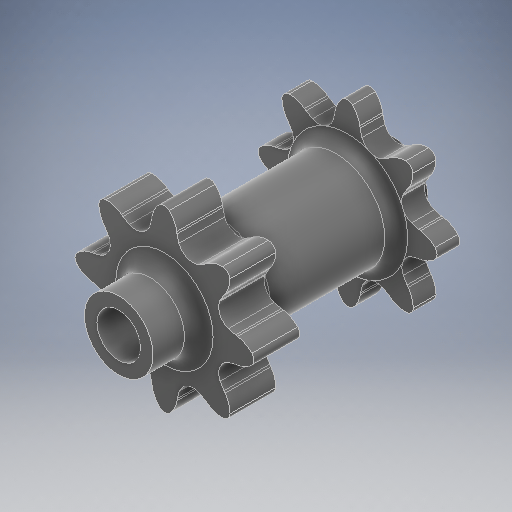
# Autodesk Inventor part: 6PSprocketElongated
Saved by Autodesk Inventor 2026.1 (Build 301233000, 233)
## iProperties
Created: 2025-10-13
Part Number: 6PSprocketElongated
Material: Plastic, Opaque Black
Document SubType Name: Modeling
Designer: Teddy
Density: 0.952 g/cm^3
Appearance: Smooth - Black
Author: Teddy
Autodesk Inventor part; units mm, degrees
ref_plane "YZ Plane" through (0, 0, 0) normal (1, 0, 0) x (0, 1, 0)
ref_plane "XZ Plane" through (0, 0, 0) normal (0, 1, 0) x (-1, 0, 0)
ref_plane "XY Plane" through (0, 0, 0) normal (0, 0, 1) x (1, 0, 0)
sketch "Sketch1" plane through (0, 0, 0) normal (0, 0, 1) x (1, 0, 0)
  spline S0 degree 3 poles (4.5605, -0.4358) (4.5398, -0.5666) (4.5107, -0.6964) (4.3363, -1.2739) (4.0837, -1.6899) (3.7565, -2.02) (3.7485, -2.028) (3.7404, -2.036) knots 0 0 0 0 0.215998 0.215998 0.980932 0.980932 1 1 1 1
  spline S1 degree 3 poles (3.7404, -2.036) (3.6739, -2.1011) (3.5927, -2.1577) (3.4009, -2.2429) (3.2878, -2.2658) (3.0745, -2.2664) (2.9612, -2.2441) (2.769, -2.1599) (2.6875, -2.1038) (2.6206, -2.039) knots 0 0 0 0 0.231931 0.231931 0.5 0.5 0.768069 0.768069 1 1 1 1
  spline S2 degree 3 poles (2.6206, -2.039) (2.6125, -2.0311) (2.6044, -2.0231) (2.2754, -1.6948) (2.0207, -1.2801) (1.8431, -0.7036) (1.8133, -0.5739) (1.7919, -0.4433) knots 0 0 0 0 0.019068 0.019068 0.784002 0.784002 1 1 1 1
  line L0 (1.7919, -0.4433) -> (1.757, -0.2271)
  spline S3 degree 3 poles (1.757, -0.2271) (1.7125, 0.0474) (1.6406, 0.3168) (1.549, 0.5685) knots 0 0 0 0 1 1 1 1
  ellipse E0 centre (-0.0213, 0.0205) end of major axis (-1.6252, 0.4958) minor radius 1.645 (1.549, 0.5685) -> (1.4956, 0.6969) ccw
  spline S4 degree 3 poles (1.4956, 0.6969) (1.4886, 0.712) (1.4813, 0.727) (1.4457, 0.7976) (1.4144, 0.852) (1.3798, 0.9048) knots 0 0 0 0 0.212597 0.212597 1 1 1 1
  arc A0 (1.3798, 0.9048) -> (-0.3446, 1.6136) centre (0, 0) ccw
  spline S5 degree 3 poles (-0.3446, 1.6136) (-0.4235, 1.5968) (-0.4998, 1.5744) (-0.5732, 1.5473) knots 0 0 0 0 1 1 1 1
  spline S6 degree 3 poles (-0.7014, 1.4935) (-0.9435, 1.3789) (-1.1841, 1.238) (-1.4088, 1.0742) knots 0 0 0 0 1 1 1 1
  ellipse E1 centre (0.0296, -0.0004) end of major axis (-1.4449, 0.7896) minor radius 1.645 (-0.5732, 1.5473) -> (-0.7014, 1.4935) ccw
  line L1 (-1.4088, 1.0742) -> (-1.5856, 0.945)
  spline S7 degree 3 poles (-1.5856, 0.945) (-1.6928, 0.8673) (-1.8052, 0.796) (-2.3368, 0.511) (-2.8095, 0.3954) (-3.2744, 0.3934) (-3.2857, 0.3934) (-3.297, 0.3935) knots 0 0 0 0 0.215998 0.215998 0.980932 0.980932 1 1 1 1
  spline S8 degree 3 poles (-3.297, 0.3935) (-3.3901, 0.3944) (-3.4875, 0.4119) (-3.6834, 0.4872) (-3.7796, 0.551) (-3.9308, 0.7015) (-3.9951, 0.7973) (-4.0715, 0.9927) (-4.0895, 1.0901) (-4.091, 1.1832) knots 0 0 0 0 0.231931 0.231931 0.5 0.5 0.768069 0.768069 1 1 1 1
  spline S9 degree 3 poles (-4.091, 1.1832) (-4.0911, 1.1945) (-4.0912, 1.2058) (-4.0917, 1.6706) (-3.9786, 2.144) (-3.6965, 2.6771) (-3.6258, 2.7899) (-3.5487, 2.8975) knots 0 0 0 0 0.019068 0.019068 0.784002 0.784002 1 1 1 1
  line L2 (-3.5487, 2.8975) -> (-3.4204, 3.075)
  spline S10 degree 3 poles (-3.4204, 3.075) (-3.2578, 3.3006) (-3.1182, 3.5419) (-3.0049, 3.7847) knots 0 0 0 0 1 1 1 1
  ellipse E2 centre (-4.5028, 4.5076) end of major axis (-5.3008, 5.9778) minor radius 1.645 (-3.0049, 3.7847) -> (-2.9519, 3.9132) ccw
  spline S11 degree 3 poles (-2.9519, 3.9132) (-2.9462, 3.9288) (-2.9407, 3.9446) (-2.9159, 4.0197) (-2.8996, 4.0803) (-2.8868, 4.1421) knots 0 0 0 0 0.212597 0.212597 1 1 1 1
  arc A1 (-2.8868, 4.1421) -> (-3.6049, 5.8627) centre (-4.5022, 4.478) ccw
  spline S12 degree 3 poles (-3.6049, 5.8627) (-3.6726, 5.9066) (-3.7424, 5.9447) (-3.8134, 5.9774) knots 0 0 0 0 1 1 1 1
  ellipse E3 centre (-4.4816, 4.4568) end of major axis (-4.9656, 6.058) minor radius 1.645 (-3.8134, 5.9774) -> (-3.9421, 6.03) ccw
  spline S13 degree 3 poles (-3.9421, 6.03) (-4.1943, 6.1202) (-4.4641, 6.1907) (-4.7388, 6.2338) knots 0 0 0 0 1 1 1 1
  line L3 (-4.7388, 6.2338) -> (-4.9552, 6.2674)
  spline S14 degree 3 poles (-4.9552, 6.2674) (-5.0859, 6.2882) (-5.2158, 6.3173) (-5.7932, 6.4917) (-6.2093, 6.7442) (-6.5394, 7.0715) (-6.5474, 7.0795) (-6.5553, 7.0876) knots 0 0 0 0 0.215998 0.215998 0.980932 0.980932 1 1 1 1
  spline S15 degree 3 poles (-6.5553, 7.0876) (-6.6205, 7.1541) (-6.677, 7.2353) (-6.7622, 7.427) (-6.7852, 7.5402) (-6.7857, 7.7535) (-6.7634, 7.8668) (-6.6793, 8.059) (-6.6232, 8.1405) (-6.5584, 8.2074) knots 0 0 0 0 0.231931 0.231931 0.5 0.5 0.768069 0.768069 1 1 1 1
  spline S16 degree 3 poles (-6.5584, 8.2074) (-6.5505, 8.2155) (-6.5425, 8.2235) (-6.2142, 8.5525) (-5.7995, 8.8073) (-5.223, 8.9848) (-5.0933, 9.0146) (-4.9627, 9.0361) knots 0 0 0 0 0.019068 0.019068 0.784002 0.784002 1 1 1 1
  line L4 (-4.9627, 9.0361) -> (-4.7465, 9.071)
  spline S17 degree 3 poles (-4.7465, 9.071) (-4.472, 9.1155) (-4.2026, 9.1874) (-3.9509, 9.279) knots 0 0 0 0 1 1 1 1
  ellipse E4 centre (-4.4988, 10.8493) end of major axis (-4.0235, 12.4532) minor radius 1.645 (-3.9509, 9.279) -> (-3.8225, 9.3324) ccw
  spline S18 degree 3 poles (-3.8225, 9.3324) (-3.7961, 9.3446) (-3.7696, 9.3578) (-3.6993, 9.3954) (-3.6564, 9.4208) (-3.6146, 9.4482) knots 0 0 0 0 0.378322 0.378322 1 1 1 1
  arc A2 (-3.6146, 9.4482) -> (-2.9058, 11.1726) centre (-4.5194, 10.828) ccw
  spline S19 degree 3 poles (-2.9058, 11.1726) (-2.9227, 11.2521) (-2.9451, 11.3283) (-2.9721, 11.4011) knots 0 0 0 0 1 1 1 1
  ellipse E5 centre (-4.5198, 10.7984) end of major axis (-3.7297, 12.2729) minor radius 1.645 (-2.9721, 11.4011) -> (-3.0258, 11.5293) ccw
  spline S20 degree 3 poles (-3.0258, 11.5293) (-3.1404, 11.7715) (-3.2813, 12.012) (-3.4451, 12.2368) knots 0 0 0 0 1 1 1 1
  line L5 (-3.4451, 12.2368) -> (-3.5743, 12.4136)
  spline S21 degree 3 poles (-3.5743, 12.4136) (-3.6521, 12.5207) (-3.7234, 12.6331) (-4.0083, 13.1648) (-4.124, 13.6375) (-4.126, 14.1023) (-4.126, 14.1136) (-4.1259, 14.125) knots 0 0 0 0 0.215998 0.215998 0.980932 0.980932 1 1 1 1
  spline S22 degree 3 poles (-4.1259, 14.125) (-4.125, 14.2181) (-4.1075, 14.3155) (-4.0321, 14.5113) (-3.9684, 14.6075) (-3.8179, 14.7588) (-3.722, 14.8231) (-3.5266, 14.8995) (-3.4293, 14.9175) (-3.3362, 14.9189) knots 0 0 0 0 0.231931 0.231931 0.5 0.5 0.768069 0.768069 1 1 1 1
  spline S23 degree 3 poles (-3.3362, 14.9189) (-3.3249, 14.9191) (-3.3136, 14.9192) (-2.8487, 14.9196) (-2.3754, 14.8066) (-1.8422, 14.5245) (-1.7294, 14.4538) (-1.6219, 14.3766) knots 0 0 0 0 0.019068 0.019068 0.784002 0.784002 1 1 1 1
  line L6 (-1.6219, 14.3766) -> (-1.4443, 14.2484)
  spline S24 degree 3 poles (-1.4443, 14.2484) (-1.2187, 14.0858) (-0.9774, 13.9462) (-0.7347, 13.8329) knots 0 0 0 0 1 1 1 1
  ellipse E6 centre (-0.0118, 15.3308) end of major axis (1.4584, 16.1288) minor radius 1.645 (-0.7347, 13.8329) -> (-0.6062, 13.7799) ccw
  spline S25 degree 3 poles (-0.6062, 13.7799) (-0.5905, 13.7742) (-0.5747, 13.7687) (-0.4996, 13.7439) (-0.439, 13.7276) (-0.3773, 13.7147) knots 0 0 0 0 0.212597 0.212597 1 1 1 1
  arc A3 (-0.3773, 13.7147) -> (1.3433, 14.4329) centre (-0.0414, 15.3302) ccw
  spline S26 degree 3 poles (1.3433, 14.4329) (1.3872, 14.5006) (1.4253, 14.5704) (1.458, 14.6414) knots 0 0 0 0 1 1 1 1
  ellipse E7 centre (-0.0626, 15.3096) end of major axis (1.5387, 15.7935) minor radius 1.645 (1.458, 14.6414) -> (1.5106, 14.7701) ccw
  spline S27 degree 3 poles (1.5106, 14.7701) (1.6008, 15.0223) (1.6713, 15.292) (1.7144, 15.5668) knots 0 0 0 0 1 1 1 1
  line L7 (1.7144, 15.5668) -> (1.7481, 15.7832)
  spline S28 degree 3 poles (1.7481, 15.7832) (1.7688, 15.9139) (1.7979, 16.0438) (1.9723, 16.6212) (2.2249, 17.0372) (2.5521, 17.3674) (2.5601, 17.3754) (2.5682, 17.3833) knots 0 0 0 0 0.215998 0.215998 0.980932 0.980932 1 1 1 1
  spline S29 degree 3 poles (2.5682, 17.3833) (2.6347, 17.4485) (2.7159, 17.505) (2.9077, 17.5902) (3.0208, 17.6131) (3.2341, 17.6137) (3.3474, 17.5914) (3.5396, 17.5072) (3.6211, 17.4511) (3.688, 17.3863) knots 0 0 0 0 0.231931 0.231931 0.5 0.5 0.768069 0.768069 1 1 1 1
  spline S30 degree 3 poles (3.688, 17.3863) (3.6961, 17.3784) (3.7042, 17.3705) (4.0332, 17.0421) (4.2879, 16.6275) (4.4655, 16.051) (4.4953, 15.9213) (4.5167, 15.7906) knots 0 0 0 0 0.019068 0.019068 0.784002 0.784002 1 1 1 1
  line L8 (4.5167, 15.7906) -> (4.5516, 15.5744)
  spline S31 degree 3 poles (4.5516, 15.5744) (4.5961, 15.2999) (4.668, 15.0306) (4.7596, 14.7788) knots 0 0 0 0 1 1 1 1
  ellipse E8 centre (6.3299, 15.3268) end of major axis (7.9338, 14.8515) minor radius 1.645 (4.7596, 14.7788) -> (4.813, 14.6505) ccw
  spline S32 degree 3 poles (4.813, 14.6505) (4.82, 14.6354) (4.8273, 14.6203) (4.8629, 14.5497) (4.8942, 14.4953) (4.9288, 14.4425) knots 0 0 0 0 0.212597 0.212597 1 1 1 1
  arc A4 (4.9288, 14.4425) -> (6.6532, 13.7337) centre (6.3086, 15.3473) ccw
  spline S33 degree 3 poles (6.6532, 13.7337) (6.7321, 13.7506) (6.8084, 13.7729) (6.8818, 13.8001) knots 0 0 0 0 1 1 1 1
  ellipse E9 centre (6.279, 15.3478) end of major axis (7.7535, 14.5577) minor radius 1.645 (6.8818, 13.8001) -> (7.01, 13.8538) ccw
  spline S34 degree 3 poles (7.01, 13.8538) (7.2521, 13.9684) (7.4927, 14.1093) (7.7174, 14.2731) knots 0 0 0 0 1 1 1 1
  line L9 (7.7174, 14.2731) -> (7.8942, 14.4023)
  spline S35 degree 3 poles (7.8942, 14.4023) (8.0014, 14.4801) (8.1138, 14.5513) (8.6454, 14.8363) (9.1181, 14.9519) (9.583, 14.954) (9.5943, 14.954) (9.6056, 14.9539) knots 0 0 0 0 0.215998 0.215998 0.980932 0.980932 1 1 1 1
  spline S36 degree 3 poles (9.6056, 14.9539) (9.6987, 14.9529) (9.7961, 14.9355) (9.992, 14.8601) (10.0882, 14.7963) (10.2394, 14.6459) (10.3037, 14.55) (10.3801, 14.3546) (10.3981, 14.2573) (10.3996, 14.1642) knots 0 0 0 0 0.231931 0.231931 0.5 0.5 0.768069 0.768069 1 1 1 1
  spline S37 degree 3 poles (10.3996, 14.1642) (10.3997, 14.1528) (10.3998, 14.1415) (10.4003, 13.6767) (10.2872, 13.2033) (10.0051, 12.6702) (9.9344, 12.5574) (9.8573, 12.4498) knots 0 0 0 0 0.019068 0.019068 0.784002 0.784002 1 1 1 1
  line L10 (9.8573, 12.4498) -> (9.729, 12.2723)
  spline S38 degree 3 poles (9.729, 12.2723) (9.5664, 12.0467) (9.4268, 11.8054) (9.3135, 11.5626) knots 0 0 0 0 1 1 1 1
  spline S39 degree 3 poles (9.3135, 11.5626) (9.2941, 11.52) (9.2763, 11.4771) (9.2605, 11.4341) knots 0 0 0 0 1 1 1 1
  spline S40 degree 3 poles (9.2605, 11.4341) (9.2548, 11.4185) (9.2493, 11.4027) (9.2245, 11.3276) (9.2082, 11.267) (9.1954, 11.2052) knots 0 0 0 0 0.212597 0.212597 1 1 1 1
  arc A5 (9.1954, 11.2052) -> (9.9135, 9.4847) centre (10.8108, 10.8693) ccw
  spline S41 degree 3 poles (9.9135, 9.4847) (9.9812, 9.4408) (10.051, 9.4026) (10.122, 9.37) knots 0 0 0 0 1 1 1 1
  ellipse E10 centre (10.7902, 10.8906) end of major axis (11.2742, 9.2893) minor radius 1.645 (10.122, 9.37) -> (10.2507, 9.3173) ccw
  spline S42 degree 3 poles (10.2507, 9.3173) (10.5029, 9.2271) (10.7727, 9.1567) (11.0474, 9.1136) knots 0 0 0 0 1 1 1 1
  line L11 (11.0474, 9.1136) -> (11.2638, 9.0799)
  spline S43 degree 3 poles (11.2638, 9.0799) (11.3945, 9.0591) (11.5244, 9.03) (12.1018, 8.8556) (12.5179, 8.6031) (12.848, 8.2759) (12.856, 8.2679) (12.8639, 8.2598) knots 0 0 0 0 0.215998 0.215998 0.980932 0.980932 1 1 1 1
  spline S44 degree 3 poles (12.8639, 8.2598) (12.9291, 8.1933) (12.9856, 8.1121) (13.0708, 7.9203) (13.0938, 7.8072) (13.0943, 7.5938) (13.072, 7.4806) (12.9879, 7.2884) (12.9318, 7.2068) (12.867, 7.14) knots 0 0 0 0 0.231931 0.231931 0.5 0.5 0.768069 0.768069 1 1 1 1
  spline S45 degree 3 poles (12.867, 7.14) (12.859, 7.1319) (12.8511, 7.1238) (12.5228, 6.7948) (12.1081, 6.54) (11.5316, 6.3625) (11.4019, 6.3327) (11.2713, 6.3112) knots 0 0 0 0 0.019068 0.019068 0.784002 0.784002 1 1 1 1
  line L12 (11.2713, 6.3112) -> (11.0551, 6.2764)
  spline S46 degree 3 poles (11.0551, 6.2764) (10.7806, 6.2318) (10.5112, 6.1599) (10.2595, 6.0683) knots 0 0 0 0 1 1 1 1
  ellipse E11 centre (10.8074, 4.498) end of major axis (10.3321, 2.8941) minor radius 1.645 (10.2595, 6.0683) -> (10.1311, 6.015) ccw
  spline S47 degree 3 poles (10.1311, 6.015) (10.116, 6.008) (10.101, 6.0007) (10.0303, 5.9651) (9.976, 5.9338) (9.9232, 5.8992) knots 0 0 0 0 0.212597 0.212597 1 1 1 1
  arc A6 (9.9232, 5.8992) -> (9.2144, 4.1748) centre (10.828, 4.5194) ccw
  spline S48 degree 3 poles (9.2144, 4.1748) (9.2312, 4.0959) (9.2536, 4.0195) (9.2807, 3.9462) knots 0 0 0 0 1 1 1 1
  ellipse E12 centre (10.8284, 4.549) end of major axis (10.0383, 3.0745) minor radius 1.645 (9.2807, 3.9462) -> (9.3344, 3.818) ccw
  spline S49 degree 3 poles (9.3344, 3.818) (9.449, 3.5759) (9.5899, 3.3353) (9.7537, 3.1106) knots 0 0 0 0 1 1 1 1
  line L13 (9.7537, 3.1106) -> (9.8829, 2.9338)
  spline S50 degree 3 poles (9.8829, 2.9338) (9.9607, 2.8266) (10.032, 2.7142) (10.3169, 2.1826) (10.4326, 1.7098) (10.4346, 1.245) (10.4346, 1.2337) (10.4345, 1.2224) knots 0 0 0 0 0.215998 0.215998 0.980932 0.980932 1 1 1 1
  spline S51 degree 3 poles (10.4345, 1.2224) (10.4336, 1.1293) (10.4161, 1.0318) (10.3407, 0.836) (10.277, 0.7398) (10.1265, 0.5885) (10.0306, 0.5242) (9.8352, 0.4478) (9.7379, 0.4298) (9.6448, 0.4284) knots 0 0 0 0 0.231931 0.231931 0.5 0.5 0.768069 0.768069 1 1 1 1
  spline S52 degree 3 poles (9.6448, 0.4284) (9.6335, 0.4283) (9.6222, 0.4282) (9.1573, 0.4277) (8.684, 0.5408) (8.1508, 0.8229) (8.038, 0.8935) (7.9305, 0.9707) knots 0 0 0 0 0.019068 0.019068 0.784002 0.784002 1 1 1 1
  line L14 (7.9305, 0.9707) -> (7.7529, 1.099)
  spline S53 degree 3 poles (7.7529, 1.099) (7.5273, 1.2615) (7.286, 1.4012) (7.0433, 1.5144) knots 0 0 0 0 1 1 1 1
  ellipse E13 centre (6.3204, 0.0166) end of major axis (4.8502, -0.7815) minor radius 1.645 (7.0433, 1.5144) -> (6.9148, 1.5675) ccw
  spline S54 degree 3 poles (6.9148, 1.5675) (6.8991, 1.5732) (6.8833, 1.5786) (6.8082, 1.6034) (6.7476, 1.6197) (6.6859, 1.6326) knots 0 0 0 0 0.212597 0.212597 1 1 1 1
  arc A7 (6.6859, 1.6326) -> (4.9653, 0.9145) centre (6.35, 0.0171) ccw
  spline S55 degree 3 poles (4.9653, 0.9145) (4.9214, 0.8468) (4.8833, 0.777) (4.8506, 0.7059) knots 0 0 0 0 1 1 1 1
  spline S56 degree 3 poles (4.8506, 0.7059) (4.8316, 0.6642) (4.814, 0.6213) (4.798, 0.5773) knots 0 0 0 0 1 1 1 1
  spline S57 degree 3 poles (4.798, 0.5773) (4.7078, 0.325) (4.6373, 0.0553) (4.5942, -0.2194) knots 0 0 0 0 1 1 1 1
  line L15 (4.5942, -0.2194) -> (4.5605, -0.4358)
  constraints: 14 other
extrude "Extrusion1" add sketch "Sketch1" against normal blind 22.86
sketch "Sketch6" plane through (0, 0, -22.86) normal (0, 0, -1) x (-1, 0, 0)
  point P0 (0, 0)
sketch "Sketch2" plane through (0, 0, 0) normal (0, 0, 1) x (1, 0, 0)
  line L0 (-0.0207, 4.4987) -> (6.3293, 4.4987)
  line L1 (6.3293, 4.4987) -> (6.3293, 10.8487)
  line L2 (6.3293, 10.8487) -> (-0.0207, 10.8487)
  line L3 (-0.0207, 10.8487) -> (-0.0207, 4.4987)
  line L4 (-0.0207, 4.4987) -> (6.3293, 10.8487) construction
  line L5 (6.3293, 4.4987) -> (-0.0207, 10.8487) construction
  line L6 (-6.5584, 8.2074) -> (-6.5553, 7.0876) construction
  line L7 (2.5682, 17.3833) -> (3.688, 17.3863) construction
  line L8 (12.8639, 8.2598) -> (12.867, 7.14) construction
  line L9 (3.7404, -2.036) -> (2.6206, -2.039) construction
  line L10 (3.1281, 17.3848) -> (3.1805, -2.0375) construction
  line L11 (-6.5569, 7.6475) -> (12.8655, 7.6999) construction
  line L12 (-1.2907, 3.2287) -> (7.5993, 3.2287)
  line L13 (7.5993, 3.2287) -> (7.5993, 12.1187)
  line L14 (7.5993, 12.1187) -> (-1.2907, 12.1187)
  line L15 (-1.2907, 12.1187) -> (-1.2907, 3.2287)
  line L16 (-1.2907, 3.2287) -> (7.5993, 12.1187) construction
  line L17 (7.5993, 3.2287) -> (-1.2907, 12.1187) construction
  circle A0 centre (3.1543, 7.6737) radius 2.413
  point P0 (0, 0)
  point P1 (3.1543, 7.6737)
  dimension "d2" = 6.35
  dimension "d3" = 6.35
  dimension "d4" = 8.89
  dimension "d5" = 8.89
  dimension "d20" = 4.826
  constraints: 36 end point, 11 midpoint, 5 perpendicular, 4 parallel, 2 horizontal, 1 centre point, 1 coincident, 4 other
  measures "d2" distance of L0.end L1.end
  measures "d3" distance of L1.end L2.end
  measures "d4" distance of L14.end L13.end
  measures "d5" distance of L12.end L13.end
  measures "d20" diameter of A0
extrude "Extrusion2" cut sketch "Sketch2" against normal through all contours A0
sketch "Sketch3" plane through (0, 0, 0) normal (0, 0, 1) x (1, 0, 0)
  circle A0 centre (3.1543, 7.6737) radius 2.413 projected
  circle A1 centre (3.1543, 7.6737) radius 2.413
  circle A2 centre (3.1543, 7.6737) radius 3.81
  dimension "d21" = 7.62
  constraints: 2 centre point, 2 coincident
  measures "d21" diameter of A2
extrude "Extrusion3" add sketch "Sketch3" along normal blind 5.08 and the other way blind 25.4
ref_plane "Work Plane1" through (0, 0, -5.08) normal (0, 0, 1) x (1, 0, 0)
fillet "Fillet1" radius 1.5875 2 edges at (-0.6557, 7.6737, 0) (-0.6557, 7.6737, -22.86)
sketch "Sketch5" plane through (0, 0, -5.08) normal (0, 0, 1) x (1, 0, 0)
  ellipse E0 centre (5.8706, 0.0084) end of major axis (6.5307, 2.2232) minor radius 1.1968 (4.798, 0.5773) -> (4.5942, -0.2194) ccw projected
  arc A0 (4.8506, 0.7059) -> (4.798, 0.5773) centre (6.4859, -0.0385) ccw projected
  arc A1 (7.0433, 1.5144) -> (4.8506, 0.7059) centre (6.35, 0.0171) ccw projected
  ellipse E1 centre (6.7074, 0.3514) end of major axis (8.735, -0.7411) minor radius 1.1905 (7.7529, 1.099) -> (7.0433, 1.5144) ccw projected
  line L0 (7.7529, 1.099) -> (7.9305, 0.9707) projected
  spline S0 degree 3 poles (7.9305, 0.9707) (8.038, 0.8935) (8.1508, 0.8229) (8.684, 0.5408) (9.1573, 0.4277) (9.6222, 0.4282) (9.6335, 0.4283) (9.6448, 0.4284) knots 0 0 0 0 0.215998 0.215998 0.980932 0.980932 1 1 1 1 projected
  spline S1 degree 3 poles (9.6448, 0.4284) (9.7379, 0.4298) (9.8352, 0.4478) (10.0306, 0.5242) (10.1265, 0.5885) (10.277, 0.7398) (10.3407, 0.836) (10.4161, 1.0318) (10.4336, 1.1293) (10.4345, 1.2224) knots 0 0 0 0 0.231931 0.231931 0.5 0.5 0.768069 0.768069 1 1 1 1 projected
  spline S2 degree 3 poles (10.4345, 1.2224) (10.4346, 1.2337) (10.4346, 1.245) (10.4326, 1.7098) (10.3169, 2.1826) (10.032, 2.7142) (9.9607, 2.8266) (9.8829, 2.9338) knots 0 0 0 0 0.019068 0.019068 0.784002 0.784002 1 1 1 1 projected
  line L1 (9.8829, 2.9338) -> (9.7537, 3.1106) projected
  ellipse E2 centre (10.4952, 4.1742) end of major axis (9.3958, 6.2071) minor radius 1.1968 (9.3344, 3.818) -> (9.7537, 3.1106) ccw projected
  arc A2 (10.2595, 6.0683) -> (9.3344, 3.818) centre (10.828, 4.5194) ccw projected
  ellipse E3 centre (10.8444, 5.0085) end of major axis (13.0506, 5.6697) minor radius 1.1905 (11.0551, 6.2764) -> (10.2595, 6.0683) ccw projected
  line L2 (11.0551, 6.2764) -> (11.2713, 6.3112) projected
  spline S3 degree 3 poles (11.2713, 6.3112) (11.4019, 6.3327) (11.5316, 6.3625) (12.1081, 6.54) (12.5228, 6.7948) (12.8511, 7.1238) (12.859, 7.1319) (12.867, 7.14) knots 0 0 0 0 0.215998 0.215998 0.980932 0.980932 1 1 1 1 projected
  spline S4 degree 3 poles (12.867, 7.14) (12.9318, 7.2068) (12.9879, 7.2884) (13.072, 7.4806) (13.0943, 7.5938) (13.0938, 7.8072) (13.0708, 7.9203) (12.9856, 8.1121) (12.9291, 8.1933) (12.8639, 8.2598) knots 0 0 0 0 0.231931 0.231931 0.5 0.5 0.768069 0.768069 1 1 1 1 projected
  spline S5 degree 3 poles (12.8639, 8.2598) (12.856, 8.2679) (12.848, 8.2759) (12.5179, 8.6031) (12.1018, 8.8556) (11.5244, 9.03) (11.3945, 9.0591) (11.2638, 9.0799) knots 0 0 0 0 0.019068 0.019068 0.784002 0.784002 1 1 1 1 projected
  line L3 (11.2638, 9.0799) -> (11.0474, 9.1136) projected
  ellipse E4 centre (10.8196, 10.39) end of major axis (13.0344, 9.7299) minor radius 1.1968 (10.2507, 9.3173) -> (11.0474, 9.1136) ccw projected
  arc A3 (9.2605, 11.4341) -> (10.2507, 9.3173) centre (10.8108, 10.8693) ccw projected
  ellipse E5 centre (10.9485, 12.0286) end of major axis (12.6047, 13.3631) minor radius 0.9794 (9.3135, 11.5626) -> (9.2605, 11.4341) ccw projected
  ellipse E6 centre (10.4766, 11.2268) end of major axis (11.5691, 13.2544) minor radius 1.1905 (9.729, 12.2723) -> (9.3135, 11.5626) ccw projected
  line L4 (9.729, 12.2723) -> (9.8573, 12.4498) projected
  spline S6 degree 3 poles (9.8573, 12.4498) (9.9344, 12.5574) (10.0051, 12.6702) (10.2872, 13.2033) (10.4003, 13.6767) (10.3998, 14.1415) (10.3997, 14.1528) (10.3996, 14.1642) knots 0 0 0 0 0.215998 0.215998 0.980932 0.980932 1 1 1 1 projected
  spline S7 degree 3 poles (10.3996, 14.1642) (10.3981, 14.2573) (10.3801, 14.3546) (10.3037, 14.55) (10.2394, 14.6459) (10.0882, 14.7963) (9.992, 14.8601) (9.7961, 14.9355) (9.6987, 14.9529) (9.6056, 14.9539) knots 0 0 0 0 0.231931 0.231931 0.5 0.5 0.768069 0.768069 1 1 1 1 projected
  spline S8 degree 3 poles (9.6056, 14.9539) (9.5943, 14.954) (9.583, 14.954) (9.1181, 14.9519) (8.6454, 14.8363) (8.1138, 14.5513) (8.0014, 14.4801) (7.8942, 14.4023) knots 0 0 0 0 0.019068 0.019068 0.784002 0.784002 1 1 1 1 projected
  line L5 (7.8942, 14.4023) -> (7.7174, 14.2731) projected
  ellipse E7 centre (6.6537, 15.0145) end of major axis (8.6866, 16.1139) minor radius 1.1968 (7.01, 13.8538) -> (7.7174, 14.2731) ccw projected
  arc A4 (4.7596, 14.7788) -> (7.01, 13.8538) centre (6.3086, 15.3473) ccw projected
  ellipse E8 centre (5.8195, 15.3637) end of major axis (5.1583, 17.57) minor radius 1.1905 (4.5516, 15.5744) -> (4.7596, 14.7788) ccw projected
  line L6 (4.5516, 15.5744) -> (4.5167, 15.7906) projected
  spline S9 degree 3 poles (4.5167, 15.7906) (4.4953, 15.9213) (4.4655, 16.051) (4.2879, 16.6275) (4.0332, 17.0421) (3.7042, 17.3705) (3.6961, 17.3784) (3.688, 17.3863) knots 0 0 0 0 0.215998 0.215998 0.980932 0.980932 1 1 1 1 projected
  spline S10 degree 3 poles (3.688, 17.3863) (3.6211, 17.4511) (3.5396, 17.5072) (3.3474, 17.5914) (3.2341, 17.6137) (3.0208, 17.6131) (2.9077, 17.5902) (2.7159, 17.505) (2.6347, 17.4485) (2.5682, 17.3833) knots 0 0 0 0 0.231931 0.231931 0.5 0.5 0.768069 0.768069 1 1 1 1 projected
  spline S11 degree 3 poles (2.5682, 17.3833) (2.5601, 17.3754) (2.5521, 17.3674) (2.2249, 17.0372) (1.9723, 16.6212) (1.7979, 16.0438) (1.7688, 15.9139) (1.7481, 15.7832) knots 0 0 0 0 0.019068 0.019068 0.784002 0.784002 1 1 1 1 projected
  line L7 (1.7481, 15.7832) -> (1.7144, 15.5668) projected
  ellipse E9 centre (0.438, 15.3389) end of major axis (1.0981, 17.5537) minor radius 1.1968 (1.5106, 14.7701) -> (1.7144, 15.5668) ccw projected
  arc A5 (-0.7347, 13.8329) -> (1.5106, 14.7701) centre (-0.0414, 15.3302) ccw projected
  ellipse E10 centre (-0.3988, 14.9959) end of major axis (1.6287, 13.9034) minor radius 1.1905 (-1.4443, 14.2484) -> (-0.7347, 13.8329) ccw projected
  line L8 (-1.4443, 14.2484) -> (-1.6219, 14.3766) projected
  spline S12 degree 3 poles (-1.6219, 14.3766) (-1.7294, 14.4538) (-1.8422, 14.5245) (-2.3754, 14.8066) (-2.8487, 14.9196) (-3.3136, 14.9192) (-3.3249, 14.9191) (-3.3362, 14.9189) knots 0 0 0 0 0.215998 0.215998 0.980932 0.980932 1 1 1 1 projected
  spline S13 degree 3 poles (-3.3362, 14.9189) (-3.4293, 14.9175) (-3.5266, 14.8995) (-3.722, 14.8231) (-3.8179, 14.7588) (-3.9684, 14.6075) (-4.0321, 14.5113) (-4.1075, 14.3155) (-4.125, 14.2181) (-4.1259, 14.125) knots 0 0 0 0 0.231931 0.231931 0.5 0.5 0.768069 0.768069 1 1 1 1 projected
  spline S14 degree 3 poles (-4.1259, 14.125) (-4.126, 14.1136) (-4.126, 14.1023) (-4.124, 13.6375) (-4.0083, 13.1648) (-3.7234, 12.6331) (-3.6521, 12.5207) (-3.5743, 12.4136) knots 0 0 0 0 0.019068 0.019068 0.784002 0.784002 1 1 1 1 projected
  line L9 (-3.5743, 12.4136) -> (-3.4451, 12.2368) projected
  ellipse E11 centre (-4.1866, 11.1731) end of major axis (-5.2859, 13.206) minor radius 1.1968 (-3.0258, 11.5293) -> (-3.4451, 12.2368) ccw projected
  ellipse E12 centre (-4.6681, 10.8171) end of major axis (-2.8762, 10.976) minor radius 1.7151 (-2.9058, 11.1726) -> (-3.0258, 11.5293) ccw projected
  arc A6 (-3.9509, 9.279) -> (-2.9058, 11.1726) centre (-4.5194, 10.828) ccw projected
  ellipse E13 centre (-4.5358, 10.3389) end of major axis (-2.3295, 11) minor radius 1.1905 (-4.7465, 9.071) -> (-3.9509, 9.279) ccw projected
  line L10 (-4.7465, 9.071) -> (-4.9627, 9.0361) projected
  spline S15 degree 3 poles (-4.9627, 9.0361) (-5.0933, 9.0146) (-5.223, 8.9848) (-5.7995, 8.8073) (-6.2142, 8.5525) (-6.5425, 8.2235) (-6.5505, 8.2155) (-6.5584, 8.2074) knots 0 0 0 0 0.215998 0.215998 0.980932 0.980932 1 1 1 1 projected
  spline S16 degree 3 poles (-6.5584, 8.2074) (-6.6232, 8.1405) (-6.6793, 8.059) (-6.7634, 7.8668) (-6.7857, 7.7535) (-6.7852, 7.5402) (-6.7622, 7.427) (-6.677, 7.2353) (-6.6205, 7.1541) (-6.5553, 7.0876) knots 0 0 0 0 0.231931 0.231931 0.5 0.5 0.768069 0.768069 1 1 1 1 projected
  spline S17 degree 3 poles (-6.5553, 7.0876) (-6.5474, 7.0795) (-6.5394, 7.0715) (-6.2093, 6.7442) (-5.7932, 6.4917) (-5.2158, 6.3173) (-5.0859, 6.2882) (-4.9552, 6.2674) knots 0 0 0 0 0.019068 0.019068 0.784002 0.784002 1 1 1 1 projected
  line L11 (-4.9552, 6.2674) -> (-4.7388, 6.2338) projected
  ellipse E14 centre (-4.511, 4.9574) end of major axis (-2.2961, 4.2973) minor radius 1.1968 (-3.9421, 6.03) -> (-4.7388, 6.2338) ccw projected
  arc A7 (-3.0049, 3.7847) -> (-3.9421, 6.03) centre (-4.5022, 4.478) ccw projected
  ellipse E15 centre (-4.168, 4.1205) end of major axis (-3.0755, 6.1481) minor radius 1.1905 (-3.4204, 3.075) -> (-3.0049, 3.7847) ccw projected
  line L12 (-3.4204, 3.075) -> (-3.5487, 2.8975) projected
  spline S18 degree 3 poles (-3.5487, 2.8975) (-3.6258, 2.7899) (-3.6965, 2.6771) (-3.9786, 2.144) (-4.0917, 1.6706) (-4.0912, 1.2058) (-4.0911, 1.1945) (-4.091, 1.1832) knots 0 0 0 0 0.215998 0.215998 0.980932 0.980932 1 1 1 1 projected
  spline S19 degree 3 poles (-4.091, 1.1832) (-4.0895, 1.0901) (-4.0715, 0.9927) (-3.9951, 0.7973) (-3.9308, 0.7015) (-3.7796, 0.551) (-3.6834, 0.4872) (-3.4875, 0.4119) (-3.3901, 0.3944) (-3.297, 0.3935) knots 0 0 0 0 0.231931 0.231931 0.5 0.5 0.768069 0.768069 1 1 1 1 projected
  spline S20 degree 3 poles (-3.297, 0.3935) (-3.2857, 0.3934) (-3.2744, 0.3934) (-2.8095, 0.3954) (-2.3368, 0.511) (-1.8052, 0.796) (-1.6928, 0.8673) (-1.5856, 0.945) knots 0 0 0 0 0.019068 0.019068 0.784002 0.784002 1 1 1 1 projected
  line L13 (-1.5856, 0.945) -> (-1.4088, 1.0742) projected
  ellipse E16 centre (-0.3451, 0.3328) end of major axis (1.6877, 1.4322) minor radius 1.1968 (-0.7014, 1.4935) -> (-1.4088, 1.0742) ccw projected
  arc A8 (1.549, 0.5685) -> (-0.7014, 1.4935) centre (0, 0) ccw projected
  ellipse E17 centre (0.4891, -0.0164) end of major axis (-0.1721, 2.1898) minor radius 1.1905 (1.757, -0.2271) -> (1.549, 0.5685) ccw projected
  line L14 (1.757, -0.2271) -> (1.7919, -0.4433) projected
  spline S21 degree 3 poles (1.7919, -0.4433) (1.8133, -0.5739) (1.8431, -0.7036) (2.0207, -1.2801) (2.2754, -1.6948) (2.6044, -2.0231) (2.6125, -2.0311) (2.6206, -2.039) knots 0 0 0 0 0.215998 0.215998 0.980932 0.980932 1 1 1 1 projected
  spline S22 degree 3 poles (2.6206, -2.039) (2.6875, -2.1038) (2.769, -2.1599) (2.9612, -2.2441) (3.0745, -2.2664) (3.2878, -2.2658) (3.4009, -2.2429) (3.5927, -2.1577) (3.6739, -2.1011) (3.7404, -2.036) knots 0 0 0 0 0.231931 0.231931 0.5 0.5 0.768069 0.768069 1 1 1 1 projected
  spline S23 degree 3 poles (3.7404, -2.036) (3.7485, -2.028) (3.7565, -2.02) (4.0837, -1.6899) (4.3363, -1.2739) (4.5107, -0.6964) (4.5398, -0.5666) (4.5605, -0.4358) knots 0 0 0 0 0.019068 0.019068 0.784002 0.784002 1 1 1 1 projected
  line L15 (4.5605, -0.4358) -> (4.5942, -0.2194) projected
  circle A9 centre (3.1543, 7.6737) radius 5.3975 projected
  constraints: 42 other
extrude "Extrusion4" cut sketch "Sketch5" against normal blind 15.24
fillet "Fillet2" radius 1.27 2 edges at (-2.2432, 7.6737, -20.32) (-2.2432, 7.6737, -5.08)
body "Solid1"
